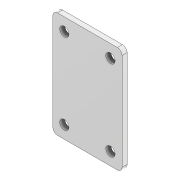
# Autodesk Inventor part: castor_support
Saved by Autodesk Inventor 2020 (Build 240168000, 168)
## iProperties
Created: 2020-09-09
Part Number: castor_support
Material: ABS 플라스틱
Document SubType Name: Modeling
Designer: 이호석
Mass: 3.09293 g
Surface Area: 30.9003 cm^2
Volume: 2.91786 cm^3
Density: 1.06 g/cm^3
Appearance: 매끄러움 - 흰색
Author: 이호석
Autodesk Inventor part; units mm, degrees
ref_plane "YZ Plane" through (0, 0, 0) normal (1, 0, 0) x (0, 1, 0)
ref_plane "XZ Plane" through (0, 0, 0) normal (0, 1, 0) x (-1, 0, 0)
ref_plane "XY Plane" through (0, 0, 0) normal (0, 0, 1) x (1, 0, 0)
sketch "스케치1" plane through (0, 0, 0) normal (0, 0, 1) x (1, 0, 0)
  line L0 (15, -23) -> (-15, -23)
  line L1 (-15, -23) -> (-15, 23)
  line L2 (-15, 23) -> (15, 23)
  line L3 (15, 23) -> (15, -23)
  circle A0 centre (-10, 17.5) radius 2
  circle A1 centre (-10, -17.5) radius 2
  circle A2 centre (10, -17.5) radius 2
  circle A3 centre (10, 17.5) radius 2
  dimension "d0" = 30
  dimension "d1" = 46
  dimension "d4" = 4
  dimension "d6" = 4
  dimension "d7" = 4
  dimension "d8" = 4
  constraints: 8 end point, 4 centre point, 2 parallel, 1 horizontal, 1 perpendicular
  measures "d0" distance of L1.end L2.end
  measures "d1" distance of L0.end L1.end
  measures "d4" diameter of A0
  measures "d6" diameter of A1
  measures "d7" diameter of A2
  measures "d8" diameter of A3
extrude "돌출1" add sketch "스케치1" along normal blind 2.2
fillet "모깎기1" radius 2 4 edges at (-15, 23, 1.1) (15, 23, 1.1) (15, -23, 1.1) (-15, -23, 1.1)
